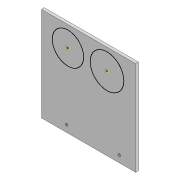
# Autodesk Inventor part: Part1
Saved by Autodesk Inventor 2020 (Build 240168000, 168)
## iProperties
Created: 2019-12-09
Part Number: Part1
Material: Generic
Document SubType Name: Modeling
Designer: Dell
Density: 1 g/cm^3
Appearance: Default
Author: Dell
Autodesk Inventor part; units mm, degrees
ref_plane "YZ Plane" through (0, 0, 0) normal (1, 0, 0) x (0, 1, 0)
ref_plane "XZ Plane" through (0, 0, 0) normal (0, 1, 0) x (-1, 0, 0)
ref_plane "XY Plane" through (0, 0, 0) normal (0, 0, 1) x (1, 0, 0)
sketch "Sketch1" plane through (0, 0, 0) normal (0, 0, 1) x (1, 0, 0)
  line L0 (0, 0) -> (200, 0)
  line L1 (200, 0) -> (200, 200)
  line L2 (200, 200) -> (0, 200)
  line L3 (0, 200) -> (0, 0)
  dimension "d0" = 200
  dimension "d1" = 200
  constraints: 8 end point, 2 parallel, 1 horizontal, 1 perpendicular
  measures "d0" distance of L2.end L1.end
  measures "d1" distance of L1.end L0.end
extrude "Extrusion1" add sketch "Sketch1" along normal blind 6
sketch "Sketch2" plane through (0, 0, 6) normal (0, 0, 1) x (1, 0, 0)
  line L0 (0, 200) -> (0, 0) projected
  circle A0 centre (55.8447, 156.8887) radius 40.7184
  circle A1 centre (158.1102, 156.8887) radius 41.3272
  circle A2 centre (55.8447, 156.8887) radius 2.5
  circle A3 centre (158.1102, 156.8887) radius 2.5
  dimension "d4" = 5
  dimension "d5" = 5
  constraints: 4 centre point, 2 coincident
  measures "d4" diameter of A2
  measures "d5" diameter of A3
extrude "Extrusion2" cut sketch "Sketch2" against normal blind 6 contours A2
sketch "Sketch3" plane through (0, 0, 6) normal (0, 0, 1) x (1, 0, 0)
  circle A0 centre (138.8739, 155.8606) radius 2.5
  point P0 (0, 0)
  dimension "d8" = 5
  constraints: 1 centre point
  measures "d8" diameter of A0
extrude "Extrusion3" cut sketch "Sketch3" against normal blind 6
sketch "Sketch4" plane through (0, 0, 6) normal (0, 0, 1) x (1, 0, 0)
  circle A0 centre (53.6423, 14.6026) radius 2.5
  point P0 (0, 0)
  dimension "d11" = 5
  constraints: 1 centre point
  measures "d11" diameter of A0
extrude "Extrusion4" cut sketch "Sketch4" against normal blind 6
sketch "Sketch5" plane through (0, 0, 6) normal (0, 0, 1) x (1, 0, 0)
  circle A0 centre (165.695, 14.6026) radius 2.5
  point P0 (0, 0)
  dimension "d14" = 5
  constraints: 1 centre point
  measures "d14" diameter of A0
extrude "Extrusion5" cut sketch "Sketch5" against normal blind 6
sketch "Sketch6" plane through (0, 0, 6) normal (0, 0, 1) x (1, 0, 0)
  circle A0 centre (55.8447, 156.8887) radius 2.5 projected
  circle A1 centre (55.8447, 156.8887) radius 33.3189
  circle A2 centre (138.8739, 155.8606) radius 2.5 projected
  circle A3 centre (138.8739, 155.8606) radius 35.7814
  point P0 (0, 0)
  constraints: 2 centre point, 2 coincident
body "Solid1"
